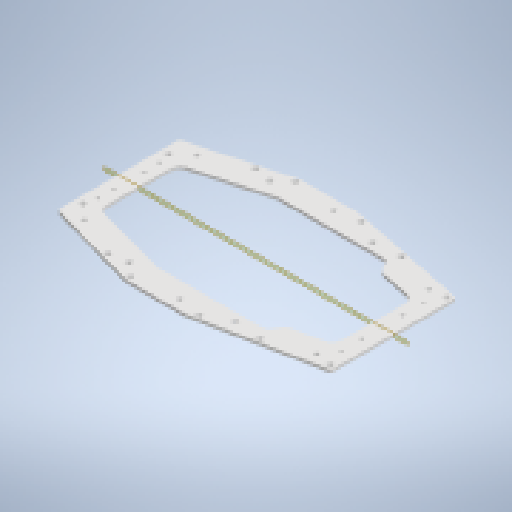
# Autodesk Inventor part: gora
Saved by Autodesk Inventor 2023.4 (Build 274418000, 418)
## iProperties
Created: 2024-06-29
Part Number: gora
Material: Ogólny
Document SubType Name: Modeling
Designer: kamil
Density: 1 g/cm^3
Appearance: Domyślna
Author: kamil
Autodesk Inventor part; units mm, degrees
ref_plane "YZ Plane" through (0, 0, 0) normal (1, 0, 0) x (0, 1, 0)
ref_plane "XZ Plane" through (0, 0, 0) normal (0, 1, 0) x (-1, 0, 0)
ref_plane "XY Plane" through (0, 0, 0) normal (0, 0, 1) x (1, 0, 0)
sketch "Szkic1" plane through (0, 0, 0) normal (0, 1, 0) x (-1, 0, 0)
  line L0 (-135, 0) -> (135, 0) construction
  line L1 (0, 75) -> (0, -75) construction
  line L2 (0, 75) -> (113.2475, 55)
  line L3 (113.2475, 55) -> (113.2475, -55)
  line L4 (113.2475, -55) -> (0, -75)
  line L5 (-113.2475, -55) -> (-113.2475, 55)
  line L6 (-113.2475, 55) -> (0, 75)
  line L7 (0, -75) -> (-113.2475, -55)
  line L8 (-113.2475, 55) -> (-135, 51.1584)
  line L9 (-135, 51.1584) -> (-135, -51.1584)
  line L10 (-135, -51.1584) -> (-113.2475, -55)
  line L11 (113.2475, 55) -> (135, 51.1584)
  line L12 (113.2475, -55) -> (135, -51.1584)
  line L13 (135, 51.1584) -> (135, -51.1584)
  line L14 (114.9866, -64.8476) -> (145, -59.5471)
  line L15 (145, -59.5471) -> (145, 59.5471)
  line L16 (145, 59.5471) -> (114.9866, 64.8476)
  line L17 (114.9866, 64.8476) -> (0, 85.1547)
  line L18 (0, 85.1547) -> (-114.9866, 64.8476)
  line L19 (-114.7917, -64.882) -> (-145, -59.5471)
  line L20 (-145, -59.5471) -> (-145, 59.5471)
  line L21 (-145, 59.5471) -> (-114.9866, 64.8476)
  line L22 (-114.7917, -64.882) -> (0, -85.1547)
  line L23 (0, -85.1547) -> (114.9866, -64.8476)
  point P0 (0, 0)
  point P1 (0, 0)
  point P2 (0, 0)
  point P3 (135, 0)
  point P4 (-135, 0)
  dimension "d0" = 270
  dimension "d1" = 115
  dimension "d2" = 115
  dimension "d3" = 115
  dimension "d4" = 115
  dimension "d5" = 150
  dimension "d6" = 110
  dimension "d7" = 10
  dimension "d8" = 10
  dimension "d9" = 10
  dimension "d10" = 10
  constraints: 48 end point, 5 vertical, 4 coincident, 4 collinear, 4 midpoint, 4 vertical alignment, 3 horizontal alignment, 1 horizontal, 6 other
  measures "d0" distance of L0.start L0.end
  measures "d1" distance of L1.start L2.end
  measures "d2" distance of L1.end L3.end
  measures "d3" distance of L1.end L5.start
  measures "d4" distance of L1.start L5.end
  measures "d5" distance of L1.end L1.start
  measures "d6" distance of L3.end L2.end
  measures "d7" distance between parallel lines of L13 L15
  measures "d8" distance between parallel lines of L2 L17
  measures "d9" distance between parallel lines of L9 L20
  measures "d10" distance between parallel lines of L7 L22
extrude "Wyciągnięcie proste1" add sketch "Szkic1" along normal blind 3 contours L2 L3 L4 L7 L5 L6 | L11 L13 L12 L3 | L5 L10 L9 L8 | L23 L22 L19 L20 L21 L18 L17 L16 L15 L14
hole "Otwór1" at (-113.2475, 0, 55) at (0, 0, 75) at (113.2475, 0, 55) at (-113.2475, 0, -55) at (0, 0, -75) at (113.2475, 0, -55) direction (0, 1, 0) diameter 3 depth 10 tip angle 118
sketch "Szkic2" plane through (0, 3, 0) normal (0, 1, 0) x (1, 0, 0)
  line L0 (-145, -59.5471) -> (0, -85.1547) projected
  line L1 (0, -85.1547) -> (145, -59.5471) projected
  line L2 (145, 59.5471) -> (0, 85.1547) projected
  line L3 (0, 85.1547) -> (-145, 59.5471) projected
  line L4 (-27.6975, -84.6887) -> (27.6975, -84.6887)
  line L5 (-26.7514, 84.6887) -> (26.7514, 84.6887)
  point P0 (0, 0)
  point P1 (0, 84.6887)
  point P2 (0, -84.6887)
  point P3 (-2.6387, 84.6887)
  point P4 (2.6387, 84.6887)
  point P5 (2.6387, -84.6887)
  point P6 (-2.6387, -84.6887)
  dimension "d20" = 0.466
  dimension "d21" = 0.466
  constraints: 4 end point, 2 horizontal, 2 midpoint, 2 vertical alignment
  measures "d20" distance from line of L4 L0.end
  measures "d21" distance from line of L5 L2.end
extrude "Wyciągnięcie proste2" cut sketch "Szkic2" against normal blind 3
sketch "Szkic3" plane through (0, 0, 0) normal (0, -1, 0) x (1, 0, 0)
  line L0 (-54, -85) -> (19, -85) projected
  line L1 (-141.3381, -18.5594) -> (-148.4685, -58.9346) projected
  line L2 (148.4685, -58.9346) -> (141.3381, -18.5594) projected
  line L3 (-54, -85) -> (-148.4685, -58.9346)
  line L4 (19, -85) -> (148.4685, -58.9346)
  line L5 (148.4685, -58.9346) -> (148.4685, 0)
  line L6 (145, 59.5471) -> (145, -59.5471) projected
  line L7 (-148.4685, -58.9346) -> (-148.4685, 0)
  line L8 (-148.4685, 0) -> (148.4685, 0)
  line L9 (-145, -59.5471) -> (-145, 59.5471) projected
  line L10 (-54, 85) -> (19, 85)
  line L11 (-54, 85) -> (-148.4685, 58.9346)
  line L12 (19, 85) -> (148.4685, 58.9346)
  line L13 (148.4685, 58.9346) -> (148.4685, 0)
  line L14 (-148.4685, 58.9346) -> (-148.4685, 0)
  line L15 (-145, 59.5471) -> (-2.6387, 84.6887) projected
  line L16 (2.6387, 84.6887) -> (145, 59.5471) projected
  line L17 (-2.6387, -84.6887) -> (-145, -59.5471) projected
  line L18 (145, -59.5471) -> (2.6387, -84.6887) projected
  line L19 (-2.6387, -84.6887) -> (2.6387, -84.6887) projected
  line L20 (2.6387, 84.6887) -> (-2.6387, 84.6887) projected
  point P0 (0, 0)
  point P1 (145, 0)
  constraints: 20 end point, 4 symmetric about line, 2 horizontal alignment, 2 vertical, 1 midpoint, 1 perpendicular
extrude "Wyciągnięcie proste3" add sketch "Szkic3" against normal blind 3 contours L3 L1 L9 L17 L19 L18 L6 L2 L4 L0 | L7 L8 L9 L1 | L2 L6 L8 L5 | L14 L11 L10 L12 L13 L8 L6 L16 L20 L15 L9
sketch "Szkic4" plane through (0, 3, 0) normal (0, 1, 0) x (1, 0, 0)
  line L0 (133.8474, 61.0533) -> (126.7423, 25.7615) projected
  line L1 (133.8474, -61.0533) -> (126.7423, -25.7615) projected
  line L2 (-134.2229, 59.5862) -> (-124.6477, 24.883) projected
  line L3 (-134.2229, -59.5862) -> (-124.6477, -24.883) projected
  line L4 (-54, 85) -> (-148.4685, 58.9346) projected
  line L5 (-148.4685, 58.9346) -> (-148.4685, -58.9346) projected
  line L6 (-148.4685, -58.9346) -> (-54, -85) projected
  line L7 (-54, -85) -> (19, -85) projected
  line L8 (19, -85) -> (148.4685, -58.9346) projected
  line L9 (148.4685, -58.9346) -> (148.4685, 58.9346) projected
  line L10 (148.4685, 58.9346) -> (19, 85) projected
  line L11 (19, 85) -> (-54, 85) projected
  circle A0 centre (0, 75) radius 1.5 projected
  circle A1 centre (113.2475, -55) radius 1.5 projected
  circle A2 centre (-113.2475, -55) radius 1.5 projected
  circle A3 centre (0, -75) radius 1.5 projected
  circle A4 centre (-113.2475, 55) radius 1.5 projected
  circle A5 centre (113.2475, 55) radius 1.5 projected
  line L12 (-134.2229, 59.5862) -> (-135.0636, 62.6332)
  line L13 (-134.2229, -59.5862) -> (-135.0636, -62.6332)
  line L14 (133.8474, 61.0533) -> (134.007, 61.846)
  line L15 (133.8474, -61.0533) -> (134.007, -61.846)
  line L16 (134.007, -61.846) -> (134.007, 61.846)
  line L17 (-135.0636, 62.6332) -> (-135.0636, -62.6332)
  point P0 (0, 0)
  constraints: 12 end point, 4 point on line, 3 collinear, 1 parallel, 1 perpendicular, 1 vertical
extrude "Wyciągnięcie proste4" cut sketch "Szkic4" against normal blind 3 contours L17 L6 L5 L4 | L10 L9 L8 L16
sketch "Szkic5" plane through (0, 0, 0) normal (0, -1, 0) x (1, 0, 0)
  line L0 (134.007, 61.846) -> (19, 85) projected
  line L1 (134.007, -61.846) -> (134.007, 61.846) projected
  line L2 (19, -85) -> (134.007, -61.846) projected
  line L3 (-54, -85) -> (19, -85) projected
  line L4 (-135.0636, -62.6332) -> (-54, -85) projected
  line L5 (-135.0636, 62.6332) -> (-135.0636, -62.6332) projected
  line L6 (-54, 85) -> (-135.0636, 62.6332) projected
  line L7 (19, 85) -> (-54, 85) projected
  line L8 (15.1367, 58.236) -> (107.007, 39.7401)
  line L9 (107.007, 39.7401) -> (107.007, -39.7401)
  line L10 (107.007, -39.7401) -> (15.1367, -58.236)
  line L11 (-51.9686, -58.236) -> (-108.7234, -42.5764)
  line L12 (-108.7234, -42.5764) -> (-108.7234, 42.5764)
  line L13 (-108.7234, 42.5764) -> (-51.9686, 58.236)
  line L14 (-17.2318, 58.236) -> (-17.2318, -58.236)
  line L15 (-17.2318, 58.236) -> (15.1367, 58.236)
  line L16 (15.1367, -58.236) -> (-17.2318, -58.236)
  line L17 (-2.2318, -43.236) -> (-2.2318, 43.236)
  line L18 (-2.2318, 43.236) -> (13.6417, 43.236)
  line L19 (13.6417, 43.236) -> (92.007, 27.459)
  line L20 (92.007, 27.459) -> (92.007, -27.459)
  line L21 (92.007, -27.459) -> (13.6417, -43.236)
  line L22 (13.6417, -43.236) -> (-2.2318, -43.236)
  line L23 (-51.9686, 58.236) -> (-17.2318, 58.236)
  line L24 (-17.2318, -58.236) -> (-51.9686, -58.236)
  line L25 (-17.2318, 43.236) -> (-49.9372, 43.236)
  line L26 (-49.9372, 43.236) -> (-93.7234, 31.1547)
  line L27 (-93.7234, 31.1547) -> (-93.7234, -31.1547)
  line L28 (-93.7234, -31.1547) -> (-49.9372, -43.236)
  line L29 (-49.9372, -43.236) -> (-17.2318, -43.236)
  line L30 (-32.2318, 70) -> (-32.2318, -70)
  point P0 (0, 0)
  point P1 (-32.2318, -43.236)
  point P2 (-32.2318, 43.236)
  dimension "d28" = 27
  dimension "d29" = 15
  dimension "d30" = 15
  dimension "d31" = 15
  constraints: 46 end point, 5 parallel, 1 horizontal, 1 perpendicular, 13 other
  measures "d28" distance between parallel lines of L0 L8
  measures "d29" distance between parallel lines of L14 L17
  measures "d30" distance between parallel lines of L23 L25
  measures "d31" distance between parallel lines of L14 L30
extrude "Wyciągnięcie proste5" cut sketch "Szkic5" against normal blind 3 contours L30 L29 L28 L27 L26 L25 | L17 L18 L19 L20 L21 L22
sketch "Szkic6" plane through (0, 3, 0) normal (0, 1, 0) x (1, 0, 0)
  line L0 (62.2834, -75.4611) -> (133.8474, -61.0533) projected
  line L1 (-135.0636, -59.3542) -> (-42.1161, -85) projected
  line L2 (62.2834, 75.4611) -> (133.8474, 61.0533) projected
  line L3 (-135.0636, 59.3542) -> (-42.1161, 85) projected
  line L4 (-54, -85) -> (19, -85) projected
  line L5 (19, -85) -> (134.007, -61.846) projected
  line L6 (62.2834, -75.4611) -> (14.903, -85)
  line L7 (134.007, 61.846) -> (19, 85) projected
  line L8 (19, 85) -> (-54, 85) projected
  line L9 (-135.0636, 62.6332) -> (-135.0636, -62.6332) projected
  line L10 (-135.0636, -62.6332) -> (-54, -85) projected
  line L11 (-54, 85) -> (-135.0636, 62.6332) projected
  line L12 (134.007, -61.846) -> (134.007, 61.846) projected
  line L13 (62.2834, 75.4611) -> (14.903, 85)
  line L14 (133.8474, 61.0533) -> (134.007, 61.0212)
  line L15 (133.8474, -61.0533) -> (134.007, -61.0212)
  point P0 (0, 0)
  constraints: 8 end point, 4 point on line, 2 collinear, 2 parallel
extrude "Wyciągnięcie proste6" cut sketch "Szkic6" against normal through all contours L0 L15 L12 L5 L4 L6 | L4 L10 L9 L1 | L14 L2 L13 L8 L7 L12 | L9 L11 L8 L3
sketch "Szkic7" plane through (0, 3, 0) normal (0, 1, 0) x (1, 0, 0)
  line L0 (13.6417, 43.236) -> (92.007, 27.459) projected
  line L1 (-2.2318, 43.236) -> (13.6417, 43.236) projected
  line L2 (-2.2318, -43.236) -> (-2.2318, 43.236) projected
  line L3 (92.007, -27.459) -> (13.6417, -43.236) projected
  line L4 (13.6417, -43.236) -> (-2.2318, -43.236) projected
  line L5 (92.007, 27.459) -> (92.007, -27.459) projected
  line L6 (-32.2318, 43.236) -> (-32.2318, -43.236) projected
  line L7 (-49.9372, 43.236) -> (-32.2318, 43.236) projected
  line L8 (-93.7234, 31.1547) -> (-49.9372, 43.236) projected
  line L9 (-93.7234, -31.1547) -> (-93.7234, 31.1547) projected
  line L10 (-49.9372, -43.236) -> (-93.7234, -31.1547) projected
  line L11 (-32.2318, -43.236) -> (-49.9372, -43.236) projected
  line L12 (-50.8456, 49.944) -> (-25.5238, 49.944)
  line L13 (-25.5238, 49.944) -> (-25.5238, -49.944)
  line L14 (-25.5238, -49.944) -> (-50.8456, -49.944)
  line L15 (-50.8456, -49.944) -> (-100.4314, -36.2625)
  line L16 (-100.4314, -36.2625) -> (-100.4314, 36.2625)
  line L17 (-100.4314, 36.2625) -> (-50.8456, 49.944)
  line L18 (14.3102, 49.944) -> (98.715, 32.9511)
  line L19 (98.715, 32.9511) -> (98.715, -32.9511)
  line L20 (98.715, -32.9511) -> (14.3102, -49.944)
  line L21 (14.3102, -49.944) -> (-8.9398, -49.944)
  line L22 (-8.9398, -49.944) -> (-8.9398, 49.944)
  line L23 (-8.9398, 49.944) -> (14.3102, 49.944)
  point P0 (0, 0)
  dimension "d36" = 6.708
  dimension "d37" = 6.708
  constraints: 24 end point, 10 other
  measures "d36" distance between parallel lines of L13 L6
  measures "d37" distance between parallel lines of L2 L22
extrude "Wyciągnięcie proste7" cut sketch "Szkic7" against normal through all contours L0 L5 L3 L4 L2 L1 | L6 L11 L10 L9 L8 L7 | L12 L13 L14 L15 L16 L17 | L18 L19 L20 L21 L22 L23
fillet "Zaokrąglenie1" radius 20 4 edges at (-42.1161, 1.5, 85) (14.903, 1.5, 85) (-42.1161, 1.5, -85) (14.903, 1.5, -85)
fillet "Zaokrąglenie2" radius 3 4 edges at (134.007, 1.5, 61.0212) (134.007, 1.5, -61.0212) (-135.0636, 1.5, 59.3542) (-135.0636, 1.5, -59.3542)
sketch "Sketch9" plane through (0, 3, 0) normal (0, 1, 0) x (1, 0, 0)
  circle A0 centre (128.7329, 56.9309) radius 2.5 projected
  circle A1 centre (72.277, 69.368) radius 2.15 projected
  circle A2 centre (46.1425, 66.8993) radius 2.15 projected
  circle A3 centre (22.9994, 79.2889) radius 2.15 projected
  circle A4 centre (-43.0005, 80.606) radius 2.15 projected
  circle A5 centre (-56.0688, 68.7013) radius 2.15 projected
  circle A6 centre (-73.3928, 72.2202) radius 2.15 projected
  circle A7 centre (-128.0641, 41.575) radius 2.15 projected
  line L0 (403.4391, -0.0004) -> (-425.8451, -0.0004)
  circle A8 centre (128.7329, -56.9317) radius 2.5
  circle A9 centre (72.277, -69.3688) radius 2.15
  circle A10 centre (46.1425, -66.9001) radius 2.15
  circle A11 centre (22.9994, -79.2897) radius 2.15
  circle A12 centre (-43.0005, -80.6068) radius 2.15
  circle A13 centre (-56.0688, -68.7021) radius 2.15
  circle A14 centre (-73.3928, -72.221) radius 2.15
  circle A15 centre (-128.0641, -41.5758) radius 2.15
  point P0 (0, 0)
  constraints: 8 centre point, 8 symmetric about line, 2 end point, 1 horizontal, 10 other
ref_plane "Work Plane1" through (12.9097, 0, 0) normal (0, 0, -1) x (-1, 0, 0)
hole "Hole2" at (128.7329, 3, -56.9309) at (72.277, 3, -69.368) at (46.1425, 3, -66.8993) at (22.9994, 3, -79.2889) at (-43.0005, 3, -80.606) at (-56.0688, 3, -68.7013) at (-73.3928, 3, -72.2202) at (-128.0641, 3, -41.575) at (-128.0641, 3, 41.5758) at (-73.3928, 3, 72.221) at (-56.0688, 3, 68.7021) at (-43.0005, 3, 80.6068) at (22.9994, 3, 79.2897) at (46.1425, 3, 66.9001) at (72.277, 3, 69.3688) at (128.7329, 3, 56.9317) direction (0, -1, 0) diameter 3.2 end through all countersink diameter 6 countersink angle 90
sketch "Sketch10" plane through (0, 3, 0) normal (0, 1, 0) x (1, 0, 0)
  circle A0 centre (72.277, -69.3688) radius 3 projected
  circle A1 centre (22.9994, -79.2897) radius 3 projected
  circle A2 centre (-56.0688, -68.7021) radius 3 projected
  circle A3 centre (-128.0641, -41.5758) radius 3 projected
  circle A4 centre (-73.3928, 72.2202) radius 3 projected
  circle A5 centre (-43.0005, 80.606) radius 3 projected
  circle A6 centre (46.1425, 66.8993) radius 3 projected
  circle A7 centre (128.7329, 56.9309) radius 3 projected
  circle A8 centre (72.277, 69.368) radius 3 projected
  circle A9 centre (22.9994, 79.2889) radius 3 projected
  circle A10 centre (-56.0688, 68.7013) radius 3 projected
  circle A11 centre (-128.0641, 41.575) radius 3 projected
  circle A12 centre (-73.3928, -72.221) radius 3 projected
  circle A13 centre (-43.0005, -80.6068) radius 3 projected
  circle A14 centre (46.1425, -66.9001) radius 3 projected
  circle A15 centre (128.7329, -56.9317) radius 3 projected
  arc A16 (-132.8615, 59.9618) -> (-135.0636, 57.0699) centre (-132.0636, 57.0699) ccw projected
  line L0 (-135.0636, 57.0699) -> (-135.0636, -57.0699) projected
  arc A17 (-135.0636, -57.0699) -> (-132.8615, -59.9618) centre (-132.0636, -57.0699) ccw projected
  line L1 (-132.8615, -59.9618) -> (-44.7271, -84.2796) projected
  arc A18 (-44.7271, -84.2796) -> (-39.4076, -85) centre (-39.4076, -65) ccw projected
  line L2 (-39.4076, -85) -> (12.9097, -85) projected
  arc A19 (12.9097, -85) -> (16.857, -84.6066) centre (12.9097, -65) ccw projected
  line L3 (16.857, -84.6066) -> (131.5991, -61.506) projected
  arc A20 (131.5991, -61.506) -> (134.007, -58.565) centre (131.007, -58.565) ccw projected
  line L4 (134.007, -58.565) -> (134.007, 58.565) projected
  arc A21 (134.007, 58.565) -> (131.5991, 61.506) centre (131.007, 58.565) ccw projected
  line L5 (131.5991, 61.506) -> (16.857, 84.6066) projected
  arc A22 (16.857, 84.6066) -> (12.9097, 85) centre (12.9097, 65) ccw projected
  line L6 (12.9097, 85) -> (-39.4076, 85) projected
  arc A23 (-39.4076, 85) -> (-44.7271, 84.2796) centre (-39.4076, 65) ccw projected
  line L7 (-44.7271, 84.2796) -> (-132.8615, 59.9618) projected
  line L8 (14.3102, -49.944) -> (-8.9398, -49.944) projected
  line L9 (-8.9398, -49.944) -> (-8.9398, 49.944) projected
  line L10 (-8.9398, 49.944) -> (14.3102, 49.944) projected
  line L11 (14.3102, 49.944) -> (98.715, 32.9511) projected
  line L12 (98.715, 32.9511) -> (98.715, -32.9511) projected
  line L13 (98.715, -32.9511) -> (14.3102, -49.944) projected
  line L14 (-50.8456, -49.944) -> (-100.4314, -36.2625) projected
  line L15 (-100.4314, -36.2625) -> (-100.4314, 36.2625) projected
  line L16 (-100.4314, 36.2625) -> (-50.8456, 49.944) projected
  line L17 (-50.8456, 49.944) -> (-25.5238, 49.944) projected
  line L18 (-25.5238, 49.944) -> (-25.5238, -49.944) projected
  line L19 (-25.5238, -49.944) -> (-50.8456, -49.944) projected
  circle A24 centre (113.2475, 55) radius 1.5 projected
  circle A25 centre (-113.2475, 55) radius 1.5 projected
  circle A26 centre (0, -75) radius 1.5 projected
  circle A27 centre (-113.2475, -55) radius 1.5 projected
  circle A28 centre (113.2475, -55) radius 1.5 projected
  circle A29 centre (0, 75) radius 1.5 projected
  arc A30 (-51.6505, -55.398) -> (-25.0527, -59.0001) centre (-25.0527, 40.9999) ccw projected
  line L20 (-129.4322, -33.9368) -> (-51.6505, -55.398) projected
  line L21 (-25.0527, -59.0001) -> (65.8368, -59.0001) projected
  arc A31 (65.8368, -59.0001) -> (70.5455, -55.6818) centre (65.8368, -54.0001) ccw projected
  line L22 (71.5412, -52.8939) -> (70.5455, -55.6818) projected
  arc A32 (72.3811, -51.4082) -> (71.5412, -52.8939) centre (76.2499, -54.5756) ccw projected
  line L23 (75.663, -47.3997) -> (72.3811, -51.4082) projected
  arc A33 (78.5449, -45.6655) -> (75.663, -47.3997) centre (79.5317, -50.5672) ccw projected
  line L24 (78.5449, -45.6655) -> (128.5118, -35.6059) projected
  arc A34 (130.9065, -37.5665) -> (128.5118, -35.6059) centre (128.9065, -37.5665) ccw projected
  line L25 (-189.5682, 0) -> (188.549, 0) projected
  line L26 (-25.5238, -49.944) -> (-25.5238, 49.944) projected
  line L27 (-25.5238, -49.944) -> (-25.5238, -58.999)
  line L28 (-8.9398, -49.944) -> (-8.9398, 49.944) projected
  line L29 (-8.9398, -49.944) -> (-8.9398, -59.0001)
  line L30 (-115.0636, -37.9013) -> (-115.0636, 0)
  line L31 (-135.0636, 57.0699) -> (-135.0636, -57.0699) projected
  line L32 (114.007, -38.5261) -> (114.007, 0)
  arc A35 (-25.0527, 59.0001) -> (-51.6505, 55.398) centre (-25.0527, -40.9999) ccw
  line L33 (-129.4322, 33.9368) -> (-51.6505, 55.398)
  line L34 (-25.0527, 59.0001) -> (65.8368, 59.0001)
  arc A36 (70.5455, 55.6818) -> (65.8368, 59.0001) centre (65.8368, 54.0001) ccw
  line L35 (71.5412, 52.8939) -> (70.5455, 55.6818)
  arc A37 (71.5412, 52.8939) -> (72.3811, 51.4082) centre (76.2499, 54.5756) ccw
  line L36 (75.663, 47.3997) -> (72.3811, 51.4082)
  arc A38 (75.663, 47.3997) -> (78.5449, 45.6655) centre (79.5317, 50.5672) ccw
  line L37 (78.5449, 45.6655) -> (128.5118, 35.6059)
  line L38 (-25.5238, 49.944) -> (-25.5238, 58.999)
  line L39 (-8.9398, 49.944) -> (-8.9398, 59.0001)
  line L40 (-115.0636, 37.9013) -> (-115.0636, 0)
  line L41 (114.007, 38.5261) -> (114.007, 0)
  point P0 (0, 0)
  dimension "d49" = 20
  dimension "d50" = 20
  constraints: 26 end point, 18 symmetric about line, 10 point on circle, 9 point on line, 4 centre point, 2 parallel, 1 perpendicular, 4 other
  measures "d49" distance between parallel lines of L30 L0
  measures "d50" distance between parallel lines of L32 L4
extrude "Extrusion8" cut sketch "Sketch10" against normal through all contours L40 L33 A35 L38 L17 L16 L15 L25 | L25 L15 L14 L19 L27 A30 L20 L30 | L8 L13 L12 L25 L32 L24 A33 L23 A32 L22 A31 L21 L29 | L39 L34 A36 L35 A37 L36 A38 L37 L41 L25 L12 L11 L10
fillet "Fillet3" radius 10 8 edges at (-8.9398, 1.5, 59.0001) (-8.9398, 1.5, -59.0001) (-25.5238, 1.5, -58.999) (-25.5238, 1.5, 58.999) (-115.0636, 1.5, 37.9013) (-115.0636, 1.5, -37.9013) (114.007, 1.5, -38.5261) (114.007, 1.5, 38.5261)
sketch "Sketch11" plane through (0, 3, 0) normal (0, 1, 0) x (1, 0, 0)
  line L0 (-135.0636, 57.0699) -> (-135.0636, -57.0699) projected
  line L1 (134.007, -58.565) -> (134.007, 58.565) projected
  line L2 (-135.0636, -57.0699) -> (-135.0636, 57.0699) projected
  line L3 (134.007, 58.565) -> (134.007, -58.565) projected
  line L4 (-135.0636, 7.5) -> (134.007, 7.5)
  line L5 (134.007, 7.5) -> (134.007, -7.5)
  line L6 (134.007, -7.5) -> (-135.0636, -7.5)
  line L7 (-135.0636, -7.5) -> (-135.0636, 7.5)
  point P0 (0, 0)
  point P1 (-135.0636, 0)
  point P2 (-135.0636, 0)
  dimension "d54" = 15
  constraints: 8 end point, 2 midpoint, 2 parallel, 2 point on line, 1 coincident, 1 horizontal, 1 perpendicular
  measures "d54" distance between parallel lines of L6 L4
extrude "Extrusion9" add sketch "Sketch11" against normal blind 3
fillet "Fillet4" radius 5 8 edges at (114.007, 1.5, 7.5) (114.007, 1.5, -7.5) (-8.9398, 1.5, 7.5) (-8.9398, 1.5, -7.5) (-25.5238, 1.5, 7.5) (-25.5238, 1.5, -7.5) (-115.0636, 1.5, 7.5) (-115.0636, 1.5, -7.5)
sketch "Sketch12" plane through (0, 3, 0) normal (0, 1, 0) x (1, 0, 0)
  line L0 (114.007, -12.5) -> (114.007, -30.3387) projected
  arc A0 (105.9807, -40.142) -> (114.007, -30.3387) centre (104.007, -30.3387) ccw projected
  line L1 (105.9807, -40.142) -> (78.5449, -45.6655) projected
  arc A1 (78.5449, -45.6655) -> (75.663, -47.3997) centre (79.5317, -50.5672) ccw projected
  line L2 (75.663, -47.3997) -> (72.3811, -51.4082) projected
  arc A2 (72.3811, -51.4082) -> (71.5412, -52.8939) centre (76.2499, -54.5756) ccw projected
  line L3 (71.5412, -52.8939) -> (70.5455, -55.6818) projected
  arc A3 (65.8368, -59.0001) -> (70.5455, -55.6818) centre (65.8368, -54.0001) ccw projected
  line L4 (65.8368, -59.0001) -> (1.0602, -59.0001) projected
  arc A4 (-8.9398, -49.0001) -> (1.0602, -59.0001) centre (1.0602, -49.0001) ccw projected
  line L5 (-8.9398, -49.0001) -> (-8.9398, -12.5) projected
  arc A5 (-3.9398, -7.5) -> (-8.9398, -12.5) centre (-3.9398, -12.5) ccw projected
  line L6 (-3.9398, -7.5) -> (109.007, -7.5) projected
  arc A6 (114.007, -12.5) -> (109.007, -7.5) centre (109.007, -12.5) ccw projected
  line L7 (-115.0636, 12.5) -> (-115.0636, 30.2868) projected
  arc A7 (-107.7234, 39.9266) -> (-115.0636, 30.2868) centre (-105.0636, 30.2868) ccw projected
  line L8 (-107.7234, 39.9266) -> (-51.6505, 55.398) projected
  arc A8 (-36.6872, 58.321) -> (-51.6505, 55.398) centre (-25.0527, -40.9999) ccw projected
  arc A9 (-25.5238, 48.3889) -> (-36.6872, 58.321) centre (-35.5238, 48.3889) ccw projected
  line L9 (-25.5238, 48.3889) -> (-25.5238, 12.5) projected
  arc A10 (-30.5238, 7.5) -> (-25.5238, 12.5) centre (-30.5238, 12.5) ccw projected
  line L10 (-30.5238, 7.5) -> (-110.0636, 7.5) projected
  arc A11 (-115.0636, 12.5) -> (-110.0636, 7.5) centre (-110.0636, 12.5) ccw projected
  line L11 (134.007, -58.565) -> (134.007, 58.565) projected
  arc A12 (134.007, 58.565) -> (131.5991, 61.506) centre (131.007, 58.565) ccw projected
  line L12 (131.5991, 61.506) -> (16.857, 84.6066) projected
  arc A13 (16.857, 84.6066) -> (12.9097, 85) centre (12.9097, 65) ccw projected
  line L13 (12.9097, 85) -> (-39.4076, 85) projected
  arc A14 (-39.4076, 85) -> (-44.7271, 84.2796) centre (-39.4076, 65) ccw projected
  line L14 (-44.7271, 84.2796) -> (-132.8615, 59.9618) projected
  arc A15 (-132.8615, 59.9618) -> (-135.0636, 57.0699) centre (-132.0636, 57.0699) ccw projected
  line L15 (-135.0636, 57.0699) -> (-135.0636, -57.0699) projected
  arc A16 (-135.0636, -57.0699) -> (-132.8615, -59.9618) centre (-132.0636, -57.0699) ccw projected
  line L16 (-132.8615, -59.9618) -> (-44.7271, -84.2796) projected
  arc A17 (-44.7271, -84.2796) -> (-39.4076, -85) centre (-39.4076, -65) ccw projected
  line L17 (-39.4076, -85) -> (12.9097, -85) projected
  arc A18 (12.9097, -85) -> (16.857, -84.6066) centre (12.9097, -65) ccw projected
  line L18 (16.857, -84.6066) -> (131.5991, -61.506) projected
  arc A19 (131.5991, -61.506) -> (134.007, -58.565) centre (131.007, -58.565) ccw projected
  line L19 (-110.0636, -7.5) -> (-30.5238, -7.5) projected
  arc A20 (-25.5238, -12.5) -> (-30.5238, -7.5) centre (-30.5238, -12.5) ccw projected
  line L20 (-25.5238, -12.5) -> (-25.5238, -48.3889) projected
  arc A21 (-36.6872, -58.321) -> (-25.5238, -48.3889) centre (-35.5238, -48.3889) ccw projected
  arc A22 (-51.6505, -55.398) -> (-36.6872, -58.321) centre (-25.0527, 40.9999) ccw projected
  line L21 (-51.6505, -55.398) -> (-107.7234, -39.9266) projected
  arc A23 (-115.0636, -30.2868) -> (-107.7234, -39.9266) centre (-105.0636, -30.2868) ccw projected
  line L22 (-115.0636, -30.2868) -> (-115.0636, -12.5) projected
  arc A24 (-110.0636, -7.5) -> (-115.0636, -12.5) centre (-110.0636, -12.5) ccw projected
  circle A25 centre (113.2475, -55) radius 1.5 projected
  circle A26 centre (-113.2475, -55) radius 1.5 projected
  circle A27 centre (0, -75) radius 1.5 projected
  circle A28 centre (128.7329, -56.9317) radius 3 projected
  circle A29 centre (46.1425, -66.9001) radius 3 projected
  circle A30 centre (-43.0005, -80.6068) radius 3 projected
  circle A31 centre (-73.3928, -72.221) radius 3 projected
  circle A32 centre (-128.0641, -41.5758) radius 3 projected
  circle A33 centre (-56.0688, -68.7021) radius 3 projected
  circle A34 centre (22.9994, -79.2897) radius 3 projected
  circle A35 centre (72.277, -69.3688) radius 3 projected
  line L23 (109.007, 7.5) -> (-3.9398, 7.5) projected
  arc A36 (-8.9398, 12.5) -> (-3.9398, 7.5) centre (-3.9398, 12.5) ccw projected
  line L24 (-8.9398, 12.5) -> (-8.9398, 49.0001) projected
  arc A37 (1.0602, 59.0001) -> (-8.9398, 49.0001) centre (1.0602, 49.0001) ccw projected
  line L25 (1.0602, 59.0001) -> (65.8368, 59.0001) projected
  arc A38 (70.5455, 55.6818) -> (65.8368, 59.0001) centre (65.8368, 54.0001) ccw projected
  line L26 (70.5455, 55.6818) -> (71.5412, 52.8939) projected
  arc A39 (71.5412, 52.8939) -> (72.3811, 51.4082) centre (76.2499, 54.5756) ccw projected
  line L27 (72.3811, 51.4082) -> (75.663, 47.3997) projected
  arc A40 (75.663, 47.3997) -> (78.5449, 45.6655) centre (79.5317, 50.5672) ccw projected
  line L28 (78.5449, 45.6655) -> (105.9807, 40.142) projected
  arc A41 (114.007, 30.3387) -> (105.9807, 40.142) centre (104.007, 30.3387) ccw projected
  line L29 (114.007, 30.3387) -> (114.007, 12.5) projected
  arc A42 (109.007, 7.5) -> (114.007, 12.5) centre (109.007, 12.5) ccw projected
  circle A43 centre (-73.3928, 72.2202) radius 3 projected
  circle A44 centre (-43.0005, 80.606) radius 3 projected
  circle A45 centre (46.1425, 66.8993) radius 3 projected
  circle A46 centre (128.7329, 56.9309) radius 3 projected
  circle A47 centre (72.277, 69.368) radius 3 projected
  circle A48 centre (22.9994, 79.2889) radius 3 projected
  circle A49 centre (-56.0688, 68.7013) radius 3 projected
  circle A50 centre (-128.0641, 41.575) radius 3 projected
  circle A51 centre (113.2475, 55) radius 1.5 projected
  circle A52 centre (-113.2475, 55) radius 1.5 projected
  circle A53 centre (0, 75) radius 1.5 projected
  line L30 (-3.9398, -7.5) -> (-30.5238, -7.5) construction
  line L31 (-110.0636, -7.5) -> (-30.5238, -7.5) construction
  line L32 (-8.9398, 12.5) -> (-8.9398, -12.5) construction
  arc A54 (-110.0636, -7.5) -> (-115.0636, -12.5) centre (-110.0636, -12.5) ccw projected
  line L33 (-115.0636, -12.5) -> (-135.0636, -12.5)
  line L34 (-110.0636, -7.5) -> (-110.0636, 7.5)
  point P0 (0, 0)
  point P1 (114.007, -21.4193)
  point P2 (134.007, 0)
  point P3 (-17.2318, 0)
  point P4 (-17.2318, -7.5)
  point P5 (-8.9398, 0)
  point P6 (-17.2318, 20)
  point P7 (-17.2318, 40)
  point P8 (-17.2318, 60)
  point P9 (-17.2318, -20)
  point P10 (-17.2318, -40)
  point P11 (-17.2318, -60)
  point P12 (2.7682, 0)
  point P13 (22.7682, 0)
  point P14 (42.7682, 0)
  point P15 (62.7682, 0)
  point P16 (82.7682, 0)
  point P17 (102.7682, 0)
  point P18 (122.7682, 0)
  point P19 (-37.2318, 0)
  point P20 (-57.2318, 0)
  point P21 (-77.2318, 0)
  point P22 (-97.2318, 0)
  point P23 (122.7682, -20)
  point P24 (122.7682, -40)
  point P25 (122.7682, 20)
  point P26 (122.7682, 40)
  point P27 (-125.0636, 0)
  point P28 (-110.0636, 0)
  point P29 (-125.0636, -12.5)
  point P30 (-125.0636, -15)
  point P31 (-125.0636, -30)
  point P32 (-125.0636, 15)
  point P33 (-125.0636, 30)
  dimension "d60" = 20
  dimension "d67" = 20
  dimension "d74" = 20
  dimension "d81" = 20
  dimension "d95" = 20
  dimension "d102" = 20
  dimension "d109" = 15
  dimension "d116" = 15
  constraints: 8 end point, 6 midpoint, 6 vertical, 3 horizontal, 2 horizontal alignment, 2 perpendicular, 2 point on line, 2 vertical alignment, 25 other
  measures "d60" distance of point (-17.232, 0) point (-17.232, 20)
  measures "d67" distance of point (-17.232, 0) point (-17.232, -20)
  measures "d74" distance of point (-17.232, 0) point (2.768, 0)
  measures "d81" distance of point (-17.232, 0) point (-37.232, 0)
  measures "d95" distance of point (122.768, 0) point (122.768, -20)
  measures "d102" distance of point (122.768, 0) point (122.768, 20)
  measures "d109" distance of point (-125.064, 0) point (-125.064, -15)
  measures "d116" distance of point (-125.064, 0) point (-125.064, 15)
hole "Hole3" at (-97.2318, 3, 0) at (-77.2318, 3, 0) at (-57.2318, 3, 0) at (-37.2318, 3, 0) at (2.7682, 3, 0) at (-17.2318, 3, 40) at (-17.2318, 3, 20) at (-17.2318, 3, 0) at (-17.2318, 3, -60) at (-17.2318, 3, -40) at (102.7682, 3, 0) at (82.7682, 3, 0) at (62.7682, 3, 0) at (42.7682, 3, 0) at (22.7682, 3, 0) at (122.7682, 3, 0) at (122.7682, 3, -40) at (122.7682, 3, 40) at (122.7682, 3, 20) at (122.7682, 3, -20) at (-125.0636, 3, -30) at (-125.0636, 3, -15) at (-125.0636, 3, 15) at (-125.0636, 3, 30) at (-17.2318, 3, -20) at (-17.2318, 3, 60) direction (0, -1, 0) diameter 3.2 end through all
chamfer "Chamfer1" distance 1 angle 45 6 edges at (-113.2475, 3, -53.5) (-113.2475, 3, 56.5) (113.2475, 3, -53.5) (113.2475, 3, 56.5) (0, 3, 76.5) (0, 3, -73.5)
sketch "Sketch15" plane through (0, 3, 0) normal (0, 1, 0) x (1, 0, 0)
  line L0 (-115.0636, -30.2868) -> (-115.0636, -12.5) projected
  line L1 (-115.0636, 12.5) -> (-115.0636, 30.2868) projected
  line L2 (-107.7234, 39.9266) -> (-51.6505, 55.398) projected
  line L3 (1.0602, 59.0001) -> (65.8368, 59.0001) projected
  line L4 (65.8368, -59.0001) -> (1.0602, -59.0001) projected
  line L5 (-51.6505, -55.398) -> (-107.7234, -39.9266) projected
  line L6 (114.007, -12.5) -> (114.007, -30.3387) projected
  line L7 (114.007, 30.3387) -> (114.007, 12.5) projected
  arc A0 (-110.0636, -7.5) -> (-115.0636, -12.5) centre (-110.0636, -12.5) ccw projected
  line L8 (-115.0636, 12.5) -> (-115.0636, -12.5)
  line L9 (114.007, -30.3387) -> (114.007, -12.5) projected
  arc A1 (109.007, 7.5) -> (114.007, 12.5) centre (109.007, 12.5) ccw projected
  line L10 (114.007, -12.5) -> (114.007, 12.5)
  line L11 (-51.6505, 55.398) -> (45.3565, 82.1638)
  arc A2 (1.0602, 59.0001) -> (-8.9398, 49.0001) centre (1.0602, 49.0001) ccw projected
  line L12 (1.0602, 59.0001) -> (-116.9099, 59.0001)
  line L13 (-107.7234, -39.9266) -> (-51.6505, -55.398) projected
  line L14 (-51.6505, -55.398) -> (0.7693, -69.8615)
  line L15 (1.0602, -59.0001) -> (-56.9459, -59.0001)
  arc A3 (-107.7234, 39.9266) -> (-115.0636, 30.2868) centre (-105.0636, 30.2868) ccw projected
  arc A4 (-115.0636, -30.2868) -> (-107.7234, -39.9266) centre (-105.0636, -30.2868) ccw projected
  line L16 (78.5449, 45.6655) -> (105.9807, 40.142) projected
  arc A5 (75.663, 47.3997) -> (78.5449, 45.6655) centre (79.5317, 50.5672) ccw projected
  line L17 (72.3811, 51.4082) -> (75.663, 47.3997) projected
  arc A6 (71.5412, 52.8939) -> (72.3811, 51.4082) centre (76.2499, 54.5756) ccw projected
  line L18 (70.5455, 55.6818) -> (71.5412, 52.8939) projected
  arc A7 (70.5455, 55.6818) -> (65.8368, 59.0001) centre (65.8368, 54.0001) ccw projected
  arc A8 (114.007, 30.3387) -> (105.9807, 40.142) centre (104.007, 30.3387) ccw projected
  arc A9 (105.9807, -40.142) -> (114.007, -30.3387) centre (104.007, -30.3387) ccw projected
  line L19 (105.9807, -40.142) -> (78.5449, -45.6655) projected
  arc A10 (78.5449, -45.6655) -> (75.663, -47.3997) centre (79.5317, -50.5672) ccw projected
  line L20 (75.663, -47.3997) -> (72.3811, -51.4082) projected
  arc A11 (65.8368, -59.0001) -> (70.5455, -55.6818) centre (65.8368, -54.0001) ccw projected
  line L21 (71.5412, -52.8939) -> (70.5455, -55.6818) projected
  arc A12 (72.3811, -51.4082) -> (71.5412, -52.8939) centre (76.2499, -54.5756) ccw projected
  circle A13 centre (-17.2318, 60) radius 1.6 projected
  circle A14 centre (-17.2318, -60) radius 1.6 projected
  point P0 (0, 0)
  point P1 (-38.5955, -59.0001)
  point P2 (-18.4808, -59.0001)
  point P3 (-15.9827, -59.0001)
  point P4 (-15.9827, 59.0001)
  point P5 (-18.4808, 59.0001)
  point P6 (-38.5955, 59.0001)
  constraints: 12 end point, 4 collinear, 2 tangent, 2 vertical
extrude "Extrusion10" cut sketch "Sketch15" against normal blind 10 contours L0 L8 L1 A3 L2 L11 L12 A13 L3 A7 L18 A6 L17 A5 L16 A8 L7 L10 L6 A9 L19 A10 L20 A12 L21 A11 L4 L15 A14 L14 L5 A4
extrude "Extrusion11" add sketch "Sketch15" against normal up to surface (3 mm away) contours L15 A14 | A13 L12 picked at (-17.7281, -59.6771) picked at (-16.758, 59.5783)
